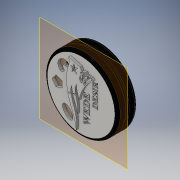
# Autodesk Inventor part: Wheel
Saved by Autodesk Inventor 2016 (Build 200138000, 138)
## iProperties
Created: 2016-10-07
Part Number: Wheel
Material: Generic
Document SubType Name: Modeling
Designer: desirw
Density: 1 g/cm^3
Appearance: Default
Mass: 52.9378 g
Surface Area: 147.304 cm^2
Volume: 52.9378 cm^3
Author: desirw
Autodesk Inventor part; units mm, degrees
ref_plane "YZ Plane" through (0, 0, 0) normal (1, 0, 0) x (0, 1, 0)
ref_plane "XZ Plane" through (0, 0, 0) normal (0, 1, 0) x (-1, 0, 0)
ref_plane "XY Plane" through (0, 0, 0) normal (0, 0, 1) x (1, 0, 0)
sketch "Sketch1" plane through (0, 0, 0) normal (0, 0, 1) x (1, 0, 0)
  circle A0 centre (0, 0) radius 31.75
  dimension "d0" = 63.5
  constraints: 1 centre point, 1 coincident
  measures "d0" diameter of A0
extrude "Extrusion1" add sketch "Sketch1" along normal blind 3.2512
sketch "Sketch2" plane through (0, 0, 3.2512) normal (0, 0, 1) x (1, 0, 0)
  circle A0 centre (0, 0) radius 33.655
  circle A1 centre (0, 0) radius 31.511
  circle A2 centre (0, 0) radius 31.511
  dimension "d3" = 67.31
  dimension "d40" = 2.144
  constraints: 3 centre point, 1 coincident
  measures "d3" diameter of A0
  measures "d40" radial gap between concentric circles of A1 A0
extrude "Extrusion2" add sketch "Sketch2" along normal blind 7.62 contours A0 | A1
sketch "Sketch3" plane through (0, 0, 0) normal (0, 0, -1) x (-1, 0, 0)
  circle A0 centre (0, 0) radius 33.655
  dimension "d6" = 67.31
  constraints: 1 centre point, 1 coincident
  measures "d6" diameter of A0
fillet "Fillet1" radius 2.54 1 edges at (-33.655, 0, 10.8712)
extrude "Extrusion3" add sketch "Sketch3" along normal blind 7.62
fillet "Fillet2" radius 2.54 1 edges at (33.655, 0, -7.62)
sketch "Sketch4" plane through (0, 0, -7.62) normal (0, 0, -1) x (-1, 0, 0)
  arc A0 (1.5256, -7.6067) -> (-1.5256, -7.6067) centre (0, -8.5367) ccw
  line L0 (1.5256, -7.6067) -> (10.0877, -14.0155)
  arc A1 (10.0877, -14.0155) -> (14.0155, -10.0877) centre (11.7691, -11.7691) ccw
  line L1 (14.0155, -10.0877) -> (7.6067, -1.5256)
  arc A2 (7.6067, 1.5256) -> (7.6067, -1.5256) centre (8.5367, 0) ccw
  line L2 (7.6067, 1.5256) -> (14.0155, 10.0877)
  arc A3 (14.0155, 10.0877) -> (10.0877, 14.0155) centre (11.7691, 11.7691) ccw
  line L3 (10.0877, 14.0155) -> (1.5256, 7.6067)
  arc A4 (-1.5256, 7.6067) -> (1.5256, 7.6067) centre (0, 8.5367) ccw
  line L4 (-1.5256, 7.6067) -> (-10.0877, 14.0155)
  arc A5 (-10.0877, 14.0155) -> (-14.0155, 10.0877) centre (-11.7691, 11.7691) ccw
  line L5 (-14.0155, 10.0877) -> (-7.6067, 1.5256)
  arc A6 (-7.6067, -1.5256) -> (-7.6067, 1.5256) centre (-8.5367, 0) ccw
  line L6 (-7.6067, -1.5256) -> (-14.0155, -10.0877)
  arc A7 (-14.0155, -10.0877) -> (-10.0877, -14.0155) centre (-11.7691, -11.7691) ccw
  line L7 (-10.0877, -14.0155) -> (-1.5256, -7.6067)
  circle A8 centre (12.339, -12.339) radius 0.75
  circle A9 centre (9.8641, -9.8641) radius 0.75
  circle A10 centre (7.3893, -7.3893) radius 0.75
  circle A11 centre (4.9144, -4.9144) radius 0.75
  circle A12 centre (12.339, 12.339) radius 0.75
  circle A13 centre (9.8641, 9.8641) radius 0.75
  circle A14 centre (7.3893, 7.3893) radius 0.75
  circle A15 centre (4.9144, 4.9144) radius 0.75
  circle A16 centre (-12.339, 12.339) radius 0.75
  circle A17 centre (-9.8641, 9.8641) radius 0.75
  circle A18 centre (-7.3893, 7.3893) radius 0.75
  circle A19 centre (-4.9144, 4.9144) radius 0.75
  circle A20 centre (-12.339, -12.339) radius 0.75
  circle A21 centre (-9.8641, -9.8641) radius 0.75
  circle A22 centre (-7.3893, -7.3893) radius 0.75
  circle A23 centre (-4.9144, -4.9144) radius 0.75
  circle A24 centre (0, 0) radius 3.6
  constraints: 25 centre point, 16 end point, 16 point on circle
extrude "Extrusion4" cut sketch "Sketch4" against normal blind 2.3622 contours A0 L7 A7 L6 A6 L5 A5 L4 A4 L3 A3 L2 A2 L1 A1 L0 | A8 | A9 | A10 | A11 | A12 | A13 | A14 | A15 | A16 | A17 | A18 | A19 | A20 | A21 | A22 | A23 | A24
sketch "Sketch5" plane through (0, 0, -7.62) normal (0, 0, -1) x (-1, 0, 0)
  circle A0 centre (0, 0) radius 3.6195
  dimension "d15" = 7.239
  constraints: 1 centre point, 1 coincident
  measures "d15" diameter of A0
extrude "Extrusion5" cut sketch "Sketch5" against normal blind 1.1684
sketch "Sketch6" plane through (0, 0, -5.2578) normal (0, 0, -1) x (-1, 0, 0)
  circle A0 centre (0, 0) radius 1.2446
  dimension "d16" = 2.4892
  constraints: 1 centre point, 1 coincident
  measures "d16" diameter of A0
extrude "Extrusion6" cut sketch "Sketch6" against normal blind 7.62
sketch "Sketch7" plane through (0, 0, 10.8712) normal (0, 0, 1) x (1, 0, 0)
  circle A0 centre (0, 0) radius 2.54
  dimension "d19" = 5.08
  constraints: 1 centre point, 1 coincident
  measures "d19" diameter of A0
extrude "Extrusion7" cut sketch "Sketch7" against normal blind 15.24
sketch "Sketch12" plane through (0, 0, -5.2578) normal (0, 0, -1) x (-1, 0, 0)
  circle A0 centre (0, 0) radius 3.5498
  circle A1 centre (0, 0) radius 3.6 projected
  dimension "d41" = 7.2
  constraints: 1 centre point, 1 coincident
  measures "d41" diameter of A1
extrude "Extrusion11" cut sketch "Sketch12" against normal blind 0.508 contours A0
sketch "Sketch13" plane through (0, 0, -7.62) normal (0, 0, -1) x (-1, 0, 0)
  circle A0 centre (-9.8641, -9.8641) radius 1.0795
  circle A1 centre (-9.8641, 9.8641) radius 1.0795
  circle A2 centre (9.8641, 9.8641) radius 1.0795
  circle A3 centre (9.8641, -9.8641) radius 1.0795
  dimension "d46" = 2.159
  dimension "d48" = 2.159
  dimension "d49" = 2.159
  dimension "d50" = 2.159
  constraints: 4 centre point
  measures "d46" diameter of A0
  measures "d48" diameter of A2
  measures "d49" diameter of A3
  measures "d50" diameter of A1
extrude "Extrusion12" cut sketch "Sketch13" against normal blind 50.8
sketch "Sketch16" plane through (0, 0, 10.8712) normal (0, 0, 1) x (1, 0, 0)
  circle A0 centre (0, 0) radius 31.115 projected
  circle A1 centre (0, 0) radius 2.54 projected
  circle A2 centre (0, 0) radius 31.115
  constraints: 1 centre point, 1 coincident, 1 concentric
extrude "Extrusion13" cut sketch "Sketch16" against normal blind 2.54
sketch "Sketch17" plane through (0, 0, 8.3312) normal (0, 0, 1) x (1, 0, 0)
  circle A0 centre (0, 0) radius 1.2446 projected
  circle A1 centre (0, 0) radius 7.62
  circle A2 centre (0, 0) radius 29.21
  dimension "d56" = 15.24
  dimension "d60" = 58.42
  constraints: 2 centre point, 2 coincident
  measures "d56" diameter of A1
  measures "d60" diameter of A2
extrude "Extrusion14" cut sketch "Sketch17" against normal blind 12.7 contours A2
fillet "Fillet3" radius 3.175 2 edges at (-29.21, 0, 8.3312) (-7.62, 0, 8.3312)
sketch "Sketch20" plane through (0, 0, -7.62) normal (0, 0, -1) x (-1, 0, 0)
  circle A0 centre (19.0012, 0) radius 8.4433
  circle A1 centre (0, 0) radius 1.2446 projected
  circle A2 centre (0, 0) radius 2.54 projected
  circle A3 centre (0, -19.0012) radius 8.4433
  circle A4 centre (-19.0012, 0) radius 8.4433
  circle A5 centre (0, 19.0012) radius 8.4433
  arc A6 (15.9108, 14.6269) -> (13.5038, 17.0339) centre (16.1061, 17.2292) ccw construction
  arc A7 (15.8105, 13.2894) -> (12.1662, 16.9336) centre (16.1061, 17.2292) ccw
  arc A8 (16.0112, 15.9644) -> (14.8413, 17.1343) centre (16.1061, 17.2292) ccw
  arc A9 (16.0112, 15.9644) -> (15.8105, 13.2894) centre (15.9108, 14.6269) ccw
  arc A10 (12.1662, 16.9336) -> (14.8413, 17.1343) centre (13.5038, 17.0339) ccw
  arc A11 (14.6269, -15.9108) -> (17.0339, -13.5038) centre (17.2292, -16.1061) ccw construction
  arc A12 (13.2894, -15.8105) -> (16.9336, -12.1662) centre (17.2292, -16.1061) ccw
  arc A13 (15.9644, -16.0112) -> (17.1343, -14.8413) centre (17.2292, -16.1061) ccw
  arc A14 (15.9644, -16.0112) -> (13.2894, -15.8105) centre (14.6269, -15.9108) ccw
  arc A15 (16.9336, -12.1662) -> (17.1343, -14.8413) centre (17.0339, -13.5038) ccw
  arc A16 (-15.9108, -14.6269) -> (-13.5038, -17.0339) centre (-16.1061, -17.2292) ccw construction
  arc A17 (-15.8105, -13.2894) -> (-12.1662, -16.9336) centre (-16.1061, -17.2292) ccw
  arc A18 (-16.0112, -15.9644) -> (-14.8413, -17.1343) centre (-16.1061, -17.2292) ccw
  arc A19 (-16.0112, -15.9644) -> (-15.8105, -13.2894) centre (-15.9108, -14.6269) ccw
  arc A20 (-12.1662, -16.9336) -> (-14.8413, -17.1343) centre (-13.5038, -17.0339) ccw
  arc A21 (-14.6269, 15.9108) -> (-17.0339, 13.5038) centre (-17.2292, 16.1061) ccw construction
  arc A22 (-13.2894, 15.8105) -> (-16.9336, 12.1662) centre (-17.2292, 16.1061) ccw
  arc A23 (-15.9644, 16.0112) -> (-17.1343, 14.8413) centre (-17.2292, 16.1061) ccw
  arc A24 (-15.9644, 16.0112) -> (-13.2894, 15.8105) centre (-14.6269, 15.9108) ccw
  arc A25 (-16.9336, 12.1662) -> (-17.1343, 14.8413) centre (-17.0339, 13.5038) ccw
  dimension "d66" = 360
  dimension "d70" = 360
  constraints: 40 point on circle, 24 centre point, 4 coincident, 4 tangent, 67 other
extrude "Extrusion15" cut sketch "Sketch20" against normal blind 10.16 contours A0 | A3 | A4 | A5 | A9 A8 A10 A7 | A14 A13 A15 A12 | A19 A18 A20 A17 | A24 A23 A25 A22
sketch "Sketch21" plane through (0, 0, -4.3688) normal (0, 0, 1) x (1, 0, 0)
  circle A0 centre (-9.8653, -9.893) radius 2.159
  circle A1 centre (-9.8653, 9.8376) radius 2.159
  circle A2 centre (9.867, -9.893) radius 2.159
  circle A3 centre (9.867, 9.8376) radius 2.159
  point P0 (0, 0)
  dimension "d74" = 4.318
  dimension "d75" = 4.318
  dimension "d76" = 4.318
  dimension "d77" = 4.318
  constraints: 4 centre point
  measures "d74" diameter of A0
  measures "d75" diameter of A1
  measures "d76" diameter of A2
  measures "d77" diameter of A3
extrude "Extrusion16" cut sketch "Sketch21" against normal blind 0.254
sketch "Sketch23" plane through (0, 0, 8.3312) normal (0, 0, 1) x (1, 0, 0)
  circle A0 centre (0, 0) radius 8.0486
  constraints: 1 centre point, 1 coincident
extrude "Extrusion17" cut sketch "Sketch23" against normal blind 12.7
ref_plane "Work Plane2" through (0, 0, 8.3312) normal (0, 0, 1) x (1, 0, 0)
sketch "Sketch24" plane through (0, 0, 8.3312) normal (0, 0, 1) x (1, 0, 0)
  circle A0 centre (0, 0) radius 31.1534
  constraints: 1 centre point, 1 coincident
extrude "Extrusion18" add sketch "Sketch24" along normal blind 2.54
sketch "Sketch25" plane through (0, 0, 10.8712) normal (0, 0, 1) x (1, 0, 0)
  line L0 (-12.7986, -29.9392) -> (-12.7986, 28.2876) construction
  line L1 (-12.7986, 28.2876) -> (14.4515, 28.2876) construction
  line L2 (14.4515, 28.2876) -> (14.4515, -29.9392) construction
  line L3 (14.4515, -29.9392) -> (-12.7986, -29.9392) construction
  arc A0 (-2.4703, -28.2892) -> (-5.6682, -15.7345) centre (-39.8581, -31.1279) ccw
  arc A1 (-10.3026, -1.9948) -> (-5.6682, -15.7345) centre (146.9864, 43.407) ccw
  arc A2 (-2.4703, -28.2892) -> (-2.4703, -18.2629) centre (-33.8456, -23.2761) ccw
  arc A3 (-2.4703, -18.2629) -> (-5.2168, -8.4433) centre (-79.7357, -34.5801) ccw
  arc A4 (-7.0459, -1.252) -> (-5.2168, -8.4433) centre (32.2007, 4.9019) ccw
  line L4 (-10.3026, -1.9948) -> (-7.0459, -1.252)
  arc A5 (-1.4091, -14.8666) -> (-3.8781, -5.8135) centre (-42.9348, -21.3286) ccw
  arc A6 (-5.6682, -0.6984) -> (-3.8781, -5.8135) centre (38.7717, 11.9828) ccw
  arc A7 (-2.9605, 0) -> (-5.6682, -0.6984) centre (0.5008, -19.0171) ccw
  arc A8 (-1.7257, -5.5998) -> (-2.9605, 0) centre (-46.1597, -12.462) ccw
  arc A9 (-1.4091, -14.8666) -> (-1.7257, -5.5998) centre (-31.0492, -11.2405) ccw
  arc A10 (13.0542, 18.6707) -> (0.223, -3.0699) centre (34.2938, -8.5214) ccw
  arc A11 (13.0542, 18.6707) -> (11.4718, 20.2531) centre (10.1474, 17.3464) ccw
  arc A12 (11.4718, 20.2531) -> (9.4266, 20.0581) centre (10.5991, 18.5838) ccw
  arc A13 (9.4266, 20.0581) -> (8.2975, 20.459) centre (7.7468, 17.1172) ccw
  arc A14 (8.2975, 20.459) -> (7.2209, 20.5419) centre (7.4283, 16.2053) ccw
  arc A15 (6.4262, 22.0118) -> (7.2209, 20.5419) centre (11.9084, 24.0263) ccw
  arc A16 (2.6562, 21.2483) -> (6.4262, 22.0118) centre (-20.9306, 147.4079) ccw
  arc A17 (2.6562, 21.2483) -> (1.1935, 24.0263) centre (-252.5291, -111.3406) ccw
  arc A18 (1.1935, 24.0263) -> (-9.4849, 27.0616) centre (-900.7825, -3128.8756) ccw
  arc A19 (-9.1238, 22.0118) -> (-9.4849, 27.0616) centre (-21.4008, 23.6716) ccw
  arc A20 (-10.3026, 17.8312) -> (-9.1238, 22.0118) centre (-36.152, 27.3765) ccw
  arc A21 (-10.3026, 17.8312) -> (-11.3285, 12.6153) centre (170.6673, -20.4736) ccw
  arc A22 (-11.3285, 12.6153) -> (-10.3026, -1.252) centre (38.6762, 9.3432) ccw
  arc A23 (-7.374, -0.5894) -> (-10.3026, -1.252) centre (0.434, -41.9034) ccw
  arc A24 (-6.6405, 5.393) -> (-7.374, -0.5894) centre (2.9307, 1.1832) ccw
  arc A25 (-6.6405, 5.393) -> (-5.8275, -0.1263) centre (42.4689, 9.8072) ccw
  arc A26 (-3.1357, 0.5919) -> (-5.8275, -0.1263) centre (0.6817, -19.118) ccw
  arc A27 (-2.2091, 8.7203) -> (-3.1357, 0.5919) centre (7.8506, 3.4565) ccw
  arc A28 (-2.2091, 8.7203) -> (-1.4091, 2.4558) centre (41.2883, 11.0914) ccw
  arc A29 (0.223, -3.0699) -> (-1.4091, 2.4558) centre (-65.3016, -19.4203) ccw
  arc A30 (6.7707, 15.7398) -> (4.847, 15.3673) centre (16.1173, -37.684) ccw
  arc A31 (4.847, 15.3673) -> (2.5284, 11.9828) centre (51.1574, -18.8455) ccw
  arc A32 (2.0647, 12.0311) -> (2.5284, 11.9828) centre (2.3182, 12.2154) ccw
  arc A33 (0.6817, 14.3084) -> (2.0647, 12.0311) centre (3.8781, 14.6909) ccw
  arc A34 (1.0059, 16.9464) -> (0.6817, 14.3084) centre (8.9448, 14.6319) ccw
  arc A35 (1.507, 17.4809) -> (1.0059, 16.9464) centre (1.5569, 16.9319) ccw
  arc A36 (1.507, 17.4809) -> (1.791, 15.7398) centre (3.5637, 16.9227) ccw
  arc A37 (1.791, 15.7398) -> (2.9878, 14.8708) centre (3.5637, 16.9227) ccw
  line L5 (2.9878, 14.8708) -> (2.9878, 18.3662)
  arc A38 (1.4604, 19.4854) -> (2.9878, 18.3662) centre (3.1078, 20.1318) ccw
  arc A39 (1.3568, 19.6561) -> (1.4604, 19.4854) centre (1.5862, 19.6786) ccw
  arc A40 (1.3568, 20.1992) -> (1.3568, 19.6561) centre (2.2724, 19.9277) ccw
  arc A41 (5.9606, 21.1505) -> (1.3568, 20.1992) centre (8.9783, -5.0691) ccw
  line L6 (5.9606, 21.1505) -> (5.9606, 18.988)
  arc A42 (5.9606, 18.988) -> (6.2957, 18.7748) centre (9.575, 24.2979) ccw
  arc A43 (6.2957, 18.7748) -> (6.9567, 19.9277) centre (-103.158, 82.2966) ccw
  arc A44 (7.5209, 19.9277) -> (6.9567, 19.9277) centre (7.2388, 19.3131) ccw
  line L7 (7.5209, 19.9277) -> (7.5209, 18.6986)
  arc A45 (8.344, 17.7097) -> (7.5209, 18.6986) centre (6.084, 16.6658) ccw
  arc A46 (8.344, 17.7097) -> (8.1842, 18.8788) centre (6.4633, 18.0481) ccw
  line L8 (8.1842, 18.8788) -> (8.1842, 20.0692)
  line L9 (8.1842, 20.0692) -> (8.4773, 20.0692)
  arc A47 (9.1501, 19.6561) -> (8.4773, 20.0692) centre (8.1291, 18.7477) ccw
  line L10 (9.1501, 19.6561) -> (9.1501, 18.878)
  arc A48 (10.3252, 19.7825) -> (9.1501, 18.878) centre (11.157, 17.4862) ccw
  line L11 (10.3252, 19.7825) -> (10.9883, 19.7825)
  arc A49 (12.0805, 18.8788) -> (10.9883, 19.7825) centre (10.1284, 17.6314) ccw
  arc A50 (12.0805, 18.8788) -> (5.0259, 10.9955) centre (36.9587, -10.4824) ccw
  arc A51 (4.3066, 11.9036) -> (5.0259, 10.9955) centre (5.7027, 12.2705) ccw
  arc A52 (4.3066, 12.6373) -> (4.3066, 11.9036) centre (5.7027, 12.2705) ccw
  arc A53 (6.7707, 15.7398) -> (4.3066, 12.6373) centre (9.0478, 11.4015) ccw
  line L12 (-3.2282, 19.8186) -> (-2.0723, 16.5796)
  line L13 (-2.0723, 16.5796) -> (-4.5876, 18.4941)
  line L14 (-4.5876, 18.4941) -> (-6.5126, 16.6185)
  line L15 (-6.5126, 16.6185) -> (-5.8751, 19.474)
  line L16 (-5.8751, 19.474) -> (-7.5613, 20.8788)
  line L17 (-7.5613, 20.8788) -> (-5.366, 21.4271)
  line L18 (-5.366, 21.4271) -> (-4.6252, 24.0672)
  line L19 (-4.6252, 24.0672) -> (-3.8073, 21.7551)
  line L20 (-3.8073, 21.7551) -> (-0.8504, 22.1353)
  line L21 (-0.8504, 22.1353) -> (-3.2282, 19.8186)
  point P0 (0, 0)
  constraints: 110 point on circle, 54 centre point, 36 end point, 5 vertical, 3 concentric, 2 point on line, 1 collinear, 1 horizontal, 1 perpendicular, 2 other
extrude "Extrusion19" add sketch "Sketch25" along normal blind 2.032
sketch "Sketch26" plane through (0, 0, 10.8712) normal (0, 0, 1) x (1, 0, 0)
  line L0 (2.4081, -21.6467) -> (2.4081, -11.4793) construction
  line L1 (2.4081, -11.4793) -> (22.0061, -11.4793) construction
  line L2 (22.0061, -11.4793) -> (22.0061, -21.6467) construction
  line L3 (22.0061, -21.6467) -> (2.4081, -21.6467) construction
  line L4 (10.6883, -4.4342) -> (10.7134, 16.181) construction
  line L5 (10.7134, 16.181) -> (15.654, 16.175) construction
  line L6 (15.654, 16.175) -> (15.6288, -4.4402) construction
  line L7 (15.6288, -4.4402) -> (10.6883, -4.4342) construction
  line L8 (2.4081, -13.0738) -> (2.5626, -13.0738)
  spline S0 degree 2 poles (2.5626, -13.0738) (2.5767, -13.233) (2.7265, -13.453) (2.8857, -13.5373) knots 0 0 0 1 2 2 2
  spline S1 degree 2 poles (2.8857, -13.5373) (2.9372, -13.5607) (3.5412, -13.7995) knots 0 0 0 1 1 1
  line L9 (3.5412, -13.7995) -> (8.2701, -15.5974)
  line L10 (8.2701, -15.5974) -> (8.2701, -15.7613)
  line L11 (8.2701, -15.7613) -> (4.5572, -17.18)
  line L12 (4.5572, -17.18) -> (8.2701, -18.7438)
  line L13 (8.2701, -18.7438) -> (8.2701, -18.8983)
  line L14 (8.2701, -18.8983) -> (3.588, -20.7852)
  spline S2 degree 2 poles (3.588, -20.7852) (2.8857, -21.0708) (2.586, -21.3002) (2.5626, -21.5718) knots 0 0 0 1 2 2 2
  line L15 (2.5626, -21.5718) -> (2.4081, -21.5718)
  line L16 (2.4081, -21.5718) -> (2.4081, -19.0902)
  line L17 (2.4081, -19.0902) -> (2.5626, -19.0902)
  spline S3 degree 2 poles (2.5626, -19.0902) (2.572, -19.3899) (2.7358, -19.5865) (2.8576, -19.5865) knots 0 0 0 1 2 2 2
  spline S4 degree 2 poles (2.8576, -19.5865) (3.0215, -19.5865) (3.5412, -19.3805) knots 0 0 0 1 1 1
  line L18 (3.5412, -19.3805) -> (6.3223, -18.2568)
  line L19 (6.3223, -18.2568) -> (4.1452, -17.3532)
  line L20 (4.1452, -17.3532) -> (3.5412, -17.5873)
  spline S5 degree 2 poles (3.5412, -17.5873) (3.0402, -17.7839) (2.7078, -17.9946) (2.5626, -18.2662) (2.5626, -18.5331) knots 0 0 0 1 2 3 3 3
  line L21 (2.5626, -18.5331) -> (2.4081, -18.5331)
  line L22 (2.4081, -18.5331) -> (2.4081, -15.7613)
  line L23 (2.4081, -15.7613) -> (2.5626, -15.7613)
  spline S6 degree 2 poles (2.5626, -15.7613) (2.5673, -16.0563) (2.6094, -16.1827) knots 0 0 0 1 1 1
  spline S7 degree 2 poles (2.6094, -16.1827) (2.6375, -16.2716) (2.778, -16.37) (2.8669, -16.37) knots 0 0 0 1 2 2 2
  spline S8 degree 2 poles (2.8669, -16.37) (2.9653, -16.37) (3.4663, -16.1827) knots 0 0 0 1 1 1
  line L24 (3.4663, -16.1827) -> (6.1772, -15.1386)
  line L25 (6.1772, -15.1386) -> (3.7238, -14.2021)
  spline S9 degree 2 poles (3.7238, -14.2021) (3.3398, -14.057) (3.0636, -13.9868) (2.9419, -13.9868) knots 0 0 0 1 2 2 2
  spline S10 degree 2 poles (2.9419, -13.9868) (2.7686, -13.9868) (2.572, -14.2256) (2.5626, -14.558) knots 0 0 0 1 2 2 2
  line L26 (2.5626, -14.558) -> (2.4081, -14.558)
  line L27 (2.4081, -14.558) -> (2.4081, -13.0738)
  line L28 (2.7358, -10.6344) -> (5.0675, -10.6344)
  line L29 (5.0675, -10.6344) -> (5.0675, -10.5173)
  spline S11 degree 2 poles (5.0675, -10.5173) (5.0675, -9.9695) (4.3839, -9.4779) (3.7144, -9.4077) knots 0 0 0 1 2 2 2
  line L30 (3.7144, -9.4077) -> (3.7144, -9.2532)
  line L31 (3.7144, -9.2532) -> (6.7156, -9.2532)
  line L32 (6.7156, -9.2532) -> (6.7156, -9.4077)
  spline S12 degree 2 poles (6.7156, -9.4077) (6.224, -9.4592) (5.6013, -9.7869) (5.3859, -10.2224) (5.3859, -10.6344) knots 0 0 0 1 2 3 3 3
  line L33 (5.3859, -10.6344) -> (7.0012, -10.6344)
  spline S13 degree 2 poles (7.0012, -10.6344) (7.4741, -10.6344) (7.6848, -10.5548) (7.8206, -10.3347) (7.8206, -10.0866) knots 0 0 0 1 2 3 3 3
  line L34 (7.8206, -10.0866) -> (7.8206, -9.7448)
  spline S14 degree 2 poles (7.8206, -9.7448) (7.8206, -8.9395) (7.0761, -7.9703) (6.3176, -7.7596) knots 0 0 0 1 2 2 2
  line L35 (6.3176, -7.7596) -> (6.3176, -7.6051)
  line L36 (6.3176, -7.6051) -> (8.139, -7.8626)
  line L37 (8.139, -7.8626) -> (8.139, -12.8162)
  line L38 (8.139, -12.8162) -> (7.9845, -12.8162)
  line L39 (7.9845, -12.8162) -> (7.9845, -12.6243)
  spline S15 degree 2 poles (7.9845, -12.6243) (7.9845, -12.3761) (7.8955, -12.2263) knots 0 0 0 1 1 1
  spline S16 degree 2 poles (7.8955, -12.2263) (7.8346, -12.1186) (7.6942, -12.0578) knots 0 0 0 1 1 1
  spline S17 degree 2 poles (7.6942, -12.0578) (7.5912, -12.0109) (7.1604, -12.0109) knots 0 0 0 1 1 1
  line L40 (7.1604, -12.0109) -> (3.3867, -12.0109)
  spline S18 degree 2 poles (3.3867, -12.0109) (2.998, -12.0109) (2.9091, -12.0297) knots 0 0 0 1 1 1
  spline S19 degree 2 poles (2.9091, -12.0297) (2.7593, -12.0765) (2.6797, -12.1888) knots 0 0 0 1 1 1
  spline S20 degree 2 poles (2.6797, -12.1888) (2.5626, -12.348) (2.5626, -12.6243) knots 0 0 0 1 1 1
  line L41 (2.5626, -12.6243) -> (2.5626, -12.8162)
  line L42 (2.5626, -12.8162) -> (2.4081, -12.8162)
  line L43 (2.4081, -12.8162) -> (2.4081, -8.0171)
  line L44 (2.4081, -8.0171) -> (4.103, -8.0171)
  line L45 (4.103, -8.0171) -> (4.103, -8.1716)
  spline S21 degree 2 poles (4.103, -8.1716) (3.4803, -8.2934) (2.9372, -8.7428) (2.8108, -9.1502) knots 0 0 0 1 2 2 2
  spline S22 degree 2 poles (2.8108, -9.1502) (2.7358, -9.3843) (2.7358, -10.0398) knots 0 0 0 1 1 1
  line L46 (2.7358, -10.0398) -> (2.7358, -10.6344)
  line L47 (8.139, -7.0994) -> (7.9845, -7.0994)
  line L48 (7.9845, -7.0994) -> (7.9845, -6.9075)
  spline S23 degree 2 poles (7.9845, -6.9075) (7.9845, -6.6593) (7.83, -6.3971) (7.6942, -6.3316) knots 0 0 0 1 2 2 2
  spline S24 degree 2 poles (7.6942, -6.3316) (7.6052, -6.2941) (7.1604, -6.2941) knots 0 0 0 1 1 1
  line L49 (7.1604, -6.2941) -> (3.3867, -6.2941)
  spline S25 degree 2 poles (3.3867, -6.2941) (2.9465, -6.2941) (2.7265, -6.3877) (2.5626, -6.6687) (2.5626, -6.9075) knots 0 0 0 1 2 3 3 3
  line L50 (2.5626, -6.9075) -> (2.5626, -7.0994)
  line L51 (2.5626, -7.0994) -> (2.4081, -7.0994)
  line L52 (2.4081, -7.0994) -> (2.4081, -4.5383)
  spline S26 degree 2 poles (2.4081, -4.5383) (2.4081, -3.5083) (2.689, -2.8855) knots 0 0 0 1 1 1
  spline S27 degree 2 poles (2.689, -2.8855) (3.0308, -2.1224) (4.4167, -1.3311) (5.2923, -1.3311) knots 0 0 0 1 2 2 2
  spline S28 degree 2 poles (5.2923, -1.3311) (5.8963, -1.3311) (6.9123, -1.7197) (7.5771, -2.3377) (7.9798, -3.1431) (8.0875, -3.7236) knots 0 0 0 1 2 3 4 4 4
  spline S29 degree 2 poles (8.0875, -3.7236) (8.139, -3.9812) (8.139, -4.5383) knots 0 0 0 1 1 1
  line L53 (8.139, -4.5383) -> (8.139, -7.0994)
  line L54 (2.7358, -4.9176) -> (7.2026, -4.9176)
  spline S30 degree 2 poles (7.2026, -4.9176) (7.5537, -4.9176) (7.7129, -4.852) (7.755, -4.7677) knots 0 0 0 1 2 2 2
  spline S31 degree 2 poles (7.755, -4.7677) (7.8206, -4.6554) (7.8206, -4.44) knots 0 0 0 1 1 1
  spline S32 degree 2 poles (7.8206, -4.44) (7.8206, -3.7377) (7.3383, -3.3631) knots 0 0 0 1 1 1
  spline S33 degree 2 poles (7.3383, -3.3631) (6.6875, -2.8575) (5.3204, -2.8575) knots 0 0 0 1 1 1
  spline S34 degree 2 poles (5.3204, -2.8575) (4.2201, -2.8575) (3.5646, -3.2039) knots 0 0 0 1 1 1
  spline S35 degree 2 poles (3.5646, -3.2039) (3.0495, -3.4802) (2.8623, -3.9109) knots 0 0 0 1 1 1
  spline S36 degree 2 poles (2.8623, -3.9109) (2.7312, -4.2106) (2.7358, -4.9176) knots 0 0 0 1 1 1
  line L55 (2.7358, 1.3892) -> (5.0675, 1.3892)
  line L56 (5.0675, 1.3892) -> (5.0675, 1.5063)
  spline S37 degree 2 poles (5.0675, 1.5063) (5.0675, 2.0541) (4.3839, 2.5457) (3.7144, 2.6159) knots 0 0 0 1 2 2 2
  line L57 (3.7144, 2.6159) -> (3.7144, 2.7704)
  line L58 (3.7144, 2.7704) -> (6.7156, 2.7704)
  line L59 (6.7156, 2.7704) -> (6.7156, 2.6159)
  spline S38 degree 2 poles (6.7156, 2.6159) (6.224, 2.5644) (5.6013, 2.2367) (5.3859, 1.8012) (5.3859, 1.3892) knots 0 0 0 1 2 3 3 3
  line L60 (5.3859, 1.3892) -> (7.0012, 1.3892)
  spline S39 degree 2 poles (7.0012, 1.3892) (7.4741, 1.3892) (7.6848, 1.4688) (7.8206, 1.6889) (7.8206, 1.937) knots 0 0 0 1 2 3 3 3
  line L61 (7.8206, 1.937) -> (7.8206, 2.2788)
  spline S40 degree 2 poles (7.8206, 2.2788) (7.8206, 3.0841) (7.0761, 4.0533) (6.3176, 4.264) knots 0 0 0 1 2 2 2
  line L62 (6.3176, 4.264) -> (6.3176, 4.4185)
  line L63 (6.3176, 4.4185) -> (8.139, 4.161)
  line L64 (8.139, 4.161) -> (8.139, -0.7926)
  line L65 (8.139, -0.7926) -> (7.9845, -0.7926)
  line L66 (7.9845, -0.7926) -> (7.9845, -0.6007)
  spline S41 degree 2 poles (7.9845, -0.6007) (7.9845, -0.3525) (7.8955, -0.2027) knots 0 0 0 1 1 1
  spline S42 degree 2 poles (7.8955, -0.2027) (7.8346, -0.095) (7.6942, -0.0342) knots 0 0 0 1 1 1
  spline S43 degree 2 poles (7.6942, -0.0342) (7.5912, 0.0127) (7.1604, 0.0127) knots 0 0 0 1 1 1
  line L67 (7.1604, 0.0127) -> (3.3867, 0.0127)
  spline S44 degree 2 poles (3.3867, 0.0127) (2.998, 0.0127) (2.9091, -0.0061) knots 0 0 0 1 1 1
  spline S45 degree 2 poles (2.9091, -0.0061) (2.7593, -0.0529) (2.6797, -0.1653) knots 0 0 0 1 1 1
  spline S46 degree 2 poles (2.6797, -0.1653) (2.5626, -0.3244) (2.5626, -0.6007) knots 0 0 0 1 1 1
  line L68 (2.5626, -0.6007) -> (2.5626, -0.7926)
  line L69 (2.5626, -0.7926) -> (2.4081, -0.7926)
  line L70 (2.4081, -0.7926) -> (2.4081, 4.0065)
  line L71 (2.4081, 4.0065) -> (4.103, 4.0065)
  line L72 (4.103, 4.0065) -> (4.103, 3.852)
  spline S47 degree 2 poles (4.103, 3.852) (3.4803, 3.7302) (2.9372, 3.2808) (2.8108, 2.8734) knots 0 0 0 1 2 2 2
  spline S48 degree 2 poles (2.8108, 2.8734) (2.7358, 2.6393) (2.7358, 1.9838) knots 0 0 0 1 1 1
  line L73 (2.7358, 1.9838) -> (2.7358, 1.3892)
  line L74 (15.5208, -4.3436) -> (15.3935, -4.3435)
  line L75 (15.3935, -4.3435) -> (15.3937, -4.1852)
  spline S49 degree 2 poles (15.3937, -4.1852) (15.3939, -3.9806) (15.2668, -3.7643) (15.1549, -3.7102) knots 0 0 0 1 2 2 2
  spline S50 degree 2 poles (15.1549, -3.7102) (15.0816, -3.6792) (14.715, -3.6787) knots 0 0 0 1 1 1
  line L76 (14.715, -3.6787) -> (11.604, -3.6749)
  spline S51 degree 2 poles (11.604, -3.6749) (11.2411, -3.6745) (11.0596, -3.7515) (10.9243, -3.9829) (10.924, -4.1797) knots 0 0 0 1 2 3 3 3
  line L77 (10.924, -4.1797) -> (10.9238, -4.338)
  line L78 (10.9238, -4.338) -> (10.7964, -4.3378)
  line L79 (10.7964, -4.3378) -> (10.799, -2.2265)
  spline S52 degree 2 poles (10.799, -2.2265) (10.8001, -1.3774) (11.0323, -0.8643) knots 0 0 0 1 1 1
  spline S53 degree 2 poles (11.0323, -0.8643) (11.3148, -0.2355) (12.4581, 0.4154) (13.1799, 0.4145) knots 0 0 0 1 2 2 2
  spline S54 degree 2 poles (13.1799, 0.4145) (13.6778, 0.4139) (14.515, 0.0925) (15.0625, -0.4176) (15.3936, -1.0819) (15.4818, -1.5606) knots 0 0 0 1 2 3 4 4 4
  spline S55 degree 2 poles (15.4818, -1.5606) (15.524, -1.773) (15.5234, -2.2323) knots 0 0 0 1 1 1
  line L80 (15.5234, -2.2323) -> (15.5208, -4.3436)
  line L81 (11.0688, -2.5395) -> (14.7511, -2.544)
  spline S56 degree 2 poles (14.7511, -2.544) (15.0406, -2.5444) (15.1719, -2.4905) (15.2067, -2.421) knots 0 0 0 1 2 2 2
  spline S57 degree 2 poles (15.2067, -2.421) (15.2608, -2.3285) (15.2611, -2.1509) knots 0 0 0 1 1 1
  spline S58 degree 2 poles (15.2611, -2.1509) (15.2618, -1.572) (14.8646, -1.2627) knots 0 0 0 1 1 1
  spline S59 degree 2 poles (14.8646, -1.2627) (14.3286, -0.8452) (13.2015, -0.8438) knots 0 0 0 1 1 1
  spline S60 degree 2 poles (13.2015, -0.8438) (12.2945, -0.8427) (11.7537, -1.1276) knots 0 0 0 1 1 1
  spline S61 degree 2 poles (11.7537, -1.1276) (11.3289, -1.3549) (11.1741, -1.7098) knots 0 0 0 1 1 1
  spline S62 degree 2 poles (11.1741, -1.7098) (11.0657, -1.9567) (11.0688, -2.5395) knots 0 0 0 1 1 1
  line L82 (11.0752, 2.6597) -> (12.9974, 2.6573)
  line L83 (12.9974, 2.6573) -> (12.9975, 2.7538)
  spline S63 degree 2 poles (12.9975, 2.7538) (12.998, 3.2054) (12.435, 3.6114) (11.8831, 3.6699) knots 0 0 0 1 2 2 2
  line L84 (11.8831, 3.6699) -> (11.8833, 3.7973)
  line L85 (11.8833, 3.7973) -> (14.3574, 3.7943)
  line L86 (14.3574, 3.7943) -> (14.3573, 3.6669)
  spline S64 degree 2 poles (14.3573, 3.6669) (13.9519, 3.6249) (13.4382, 3.3554) (13.2602, 2.9966) (13.2598, 2.657) knots 0 0 0 1 2 3 3 3
  line L87 (13.2598, 2.657) -> (14.5915, 2.6554)
  spline S65 degree 2 poles (14.5915, 2.6554) (14.9813, 2.6549) (15.1551, 2.7203) (15.2672, 2.9016) (15.2675, 3.1061) knots 0 0 0 1 2 3 3 3
  line L88 (15.2675, 3.1061) -> (15.2678, 3.3879)
  spline S66 degree 2 poles (15.2678, 3.3879) (15.2686, 4.0518) (14.6559, 4.8515) (14.0308, 5.026) knots 0 0 0 1 2 2 2
  line L89 (14.0308, 5.026) -> (14.031, 5.1533)
  line L90 (14.031, 5.1533) -> (15.5322, 4.9392)
  line L91 (15.5322, 4.9392) -> (15.5272, 0.8555)
  line L92 (15.5272, 0.8555) -> (15.3998, 0.8557)
  line L93 (15.3998, 0.8557) -> (15.4, 1.0139)
  spline S67 degree 2 poles (15.4, 1.0139) (15.4003, 1.2185) (15.3271, 1.3421) knots 0 0 0 1 1 1
  spline S68 degree 2 poles (15.3271, 1.3421) (15.277, 1.431) (15.1613, 1.4813) knots 0 0 0 1 1 1
  spline S69 degree 2 poles (15.1613, 1.4813) (15.0764, 1.52) (14.7213, 1.5204) knots 0 0 0 1 1 1
  line L94 (14.7213, 1.5204) -> (11.6103, 1.5242)
  spline S70 degree 2 poles (11.6103, 1.5242) (11.2899, 1.5246) (11.2166, 1.5093) knots 0 0 0 1 1 1
  spline S71 degree 2 poles (11.2166, 1.5093) (11.093, 1.4708) (11.0273, 1.3783) knots 0 0 0 1 1 1
  spline S72 degree 2 poles (11.0273, 1.3783) (10.9306, 1.2471) (10.9304, 1.0194) knots 0 0 0 1 1 1
  line L95 (10.9304, 1.0194) -> (10.9302, 0.8612)
  line L96 (10.9302, 0.8612) -> (10.8028, 0.8613)
  line L97 (10.8028, 0.8613) -> (10.8076, 4.8176)
  line L98 (10.8076, 4.8176) -> (12.2049, 4.8159)
  line L99 (12.2049, 4.8159) -> (12.2047, 4.6885)
  spline S73 degree 2 poles (12.2047, 4.6885) (11.6913, 4.5888) (11.2431, 4.2188) (11.1384, 3.8831) knots 0 0 0 1 2 2 2
  spline S74 degree 2 poles (11.1384, 3.8831) (11.0764, 3.6902) (11.0758, 3.1498) knots 0 0 0 1 1 1
  line L100 (11.0758, 3.1498) -> (11.0752, 2.6597)
  line L101 (10.7045, 8.8281) -> (12.2793, 8.8647)
  line L102 (12.2793, 8.8647) -> (12.2791, 8.7219)
  spline S75 degree 2 poles (12.2791, 8.7219) (11.6885, 8.6223) (10.9657, 7.8281) (10.9651, 7.3687) knots 0 0 0 1 2 2 2
  spline S76 degree 2 poles (10.9651, 7.3687) (10.9647, 7.0136) (11.3425, 6.5963) (11.5895, 6.596) knots 0 0 0 1 2 2 2
  spline S77 degree 2 poles (11.5895, 6.596) (11.7477, 6.5958) (11.8675, 6.669) knots 0 0 0 1 1 1
  spline S78 degree 2 poles (11.8675, 6.669) (12.0336, 6.7692) (12.1921, 6.9928) knots 0 0 0 1 1 1
  spline S79 degree 2 poles (12.1921, 6.9928) (12.3081, 7.1587) (12.6022, 7.7527) knots 0 0 0 1 1 1
  spline S80 degree 2 poles (12.6022, 7.7527) (13.0085, 8.5821) (13.3716, 8.8711) knots 0 0 0 1 1 1
  spline S81 degree 2 poles (13.3716, 8.8711) (13.7348, 9.1563) (14.2018, 9.1557) knots 0 0 0 1 1 1
  spline S82 degree 2 poles (14.2018, 9.1557) (14.7924, 9.155) (15.6443, 8.2315) (15.6434, 7.5174) knots 0 0 0 1 2 2 2
  spline S83 degree 2 poles (15.6434, 7.5174) (15.6431, 7.2936) (15.5539, 6.8961) (15.4261, 6.5991) knots 0 0 0 1 2 2 2
  spline S84 degree 2 poles (15.4261, 6.5991) (15.3565, 6.4293) (15.3563, 6.3212) knots 0 0 0 1 1 1
  spline S85 degree 2 poles (15.3563, 6.3212) (15.3562, 6.2325) (15.4988, 6.0277) (15.6415, 5.9658) knots 0 0 0 1 2 2 2
  line L103 (15.6415, 5.9658) -> (15.6414, 5.8384)
  line L104 (15.6414, 5.8384) -> (13.8581, 5.8406)
  line L105 (13.8581, 5.8406) -> (13.8583, 5.968)
  spline S86 degree 2 poles (13.8583, 5.968) (14.6111, 6.1214) (15.3996, 6.9966) (15.4002, 7.5023) knots 0 0 0 1 2 2 2
  spline S87 degree 2 poles (15.4002, 7.5023) (15.4007, 7.8921) (14.9767, 8.3558) (14.6949, 8.3562) knots 0 0 0 1 2 2 2
  spline S88 degree 2 poles (14.6949, 8.3562) (14.529, 8.3564) (14.2122, 8.1792) (13.93, 7.8167) (13.7056, 7.3538) knots 0 0 0 1 2 3 3 3
  spline S89 degree 2 poles (13.7056, 7.3538) (13.3883, 6.7096) (12.9399, 6.1466) (12.3914, 5.8462) (12.0595, 5.8466) knots 0 0 0 1 2 3 3 3
  spline S90 degree 2 poles (12.0595, 5.8466) (11.4959, 5.8473) (10.7018, 6.6782) (10.7026, 7.3073) knots 0 0 0 1 2 2 2
  spline S91 degree 2 poles (10.7026, 7.3073) (10.7029, 7.5389) (10.7572, 7.755) knots 0 0 0 1 1 1
  spline S92 degree 2 poles (10.7572, 7.755) (10.7998, 7.917) (11.0281, 8.3877) (11.0283, 8.4842) knots 0 0 0 1 2 2 2
  spline S93 degree 2 poles (11.0283, 8.4842) (11.0284, 8.5729) (10.9166, 8.6773) (10.7043, 8.7239) knots 0 0 0 1 2 2 2
  line L106 (10.7043, 8.7239) -> (10.7045, 8.8281)
  line L107 (15.4135, 12.0453) -> (15.5409, 12.0451)
  line L108 (15.5409, 12.0451) -> (15.5379, 9.5826)
  line L109 (15.5379, 9.5826) -> (15.4105, 9.5827)
  line L110 (15.4105, 9.5827) -> (15.4107, 9.741)
  spline S94 degree 2 poles (15.4107, 9.741) (15.4109, 9.9455) (15.3377, 10.0691) knots 0 0 0 1 1 1
  spline S95 degree 2 poles (15.3377, 10.0691) (15.2877, 10.158) (15.1719, 10.2083) knots 0 0 0 1 1 1
  spline S96 degree 2 poles (15.1719, 10.2083) (15.0871, 10.247) (14.732, 10.2474) knots 0 0 0 1 1 1
  line L111 (14.732, 10.2474) -> (11.621, 10.2512)
  spline S97 degree 2 poles (11.621, 10.2512) (11.2582, 10.2517) (11.0766, 10.1747) (10.9413, 9.9433) (10.941, 9.7464) knots 0 0 0 1 2 3 3 3
  line L112 (10.941, 9.7464) -> (10.9408, 9.5882)
  line L113 (10.9408, 9.5882) -> (10.8135, 9.5883)
  line L114 (10.8135, 9.5883) -> (10.8165, 12.0509)
  line L115 (10.8165, 12.0509) -> (10.9438, 12.0507)
  line L116 (10.9438, 12.0507) -> (10.9437, 11.8963)
  spline S98 degree 2 poles (10.9437, 11.8963) (10.9434, 11.6918) (11.0166, 11.5682) knots 0 0 0 1 1 1
  spline S99 degree 2 poles (11.0166, 11.5682) (11.0667, 11.4755) (11.1824, 11.4251) knots 0 0 0 1 1 1
  spline S100 degree 2 poles (11.1824, 11.4251) (11.2673, 11.3864) (11.6224, 11.386) knots 0 0 0 1 1 1
  line L117 (11.6224, 11.386) -> (14.7334, 11.3822)
  spline S101 degree 2 poles (14.7334, 11.3822) (15.0962, 11.3818) (15.2777, 11.4626) (15.4131, 11.694) (15.4133, 11.8909) knots 0 0 0 1 2 3 3 3
  line L118 (15.4133, 11.8909) -> (15.4135, 12.0453)
  line L119 (13.3896, 14.1166) -> (14.7135, 14.115)
  spline S102 degree 2 poles (14.7135, 14.115) (15.0995, 14.1145) (15.2965, 14.2069) (15.4164, 14.4461) (15.4168, 14.7703) knots 0 0 0 1 2 3 3 3
  line L120 (15.4168, 14.7703) -> (15.5442, 14.7701)
  line L121 (15.5442, 14.7701) -> (15.5412, 12.35)
  line L122 (15.5412, 12.35) -> (15.4139, 12.3502)
  spline S103 degree 2 poles (15.4139, 12.3502) (15.4143, 12.6783) (15.291, 12.9139) (15.0982, 13.0067) (14.7122, 13.0072) knots 0 0 0 1 2 3 3 3
  line L123 (14.7122, 13.0072) -> (11.6475, 13.011)
  spline S104 degree 2 poles (11.6475, 13.011) (11.2615, 13.0114) (11.0646, 12.919) (10.9446, 12.6799) (10.9442, 12.3556) knots 0 0 0 1 2 3 3 3
  line L124 (10.9442, 12.3556) -> (10.8168, 12.3558)
  line L125 (10.8168, 12.3558) -> (10.8195, 14.552)
  spline S105 degree 2 poles (10.8195, 14.552) (10.8206, 15.4089) (11.057, 16.2037) (11.6945, 16.7047) (12.1229, 16.7042) knots 0 0 0 1 2 3 3 3
  spline S106 degree 2 poles (12.1229, 16.7042) (12.6478, 16.7036) (12.987, 16.3249) knots 0 0 0 1 1 1
  spline S107 degree 2 poles (12.987, 16.3249) (13.2029, 16.0853) (13.3104, 15.6529) knots 0 0 0 1 1 1
  line L126 (13.3104, 15.6529) -> (14.9137, 16.7857)
  spline S108 degree 2 poles (14.9137, 16.7857) (15.2266, 17.0092) (15.3, 17.1056) knots 0 0 0 1 1 1
  spline S109 degree 2 poles (15.3, 17.1056) (15.4083, 17.2483) (15.4201, 17.4374) knots 0 0 0 1 1 1
  line L127 (15.4201, 17.4374) -> (15.5475, 17.4372)
  line L128 (15.5475, 17.4372) -> (15.5456, 15.9474)
  line L129 (15.5456, 15.9474) -> (13.39, 14.4254)
  line L130 (13.39, 14.4254) -> (13.3896, 14.1166)
  line L131 (11.0737, 14.1194) -> (13.1426, 14.1169)
  line L132 (13.1426, 14.1169) -> (13.1428, 14.3137)
  spline S110 degree 2 poles (13.1428, 14.3137) (13.1434, 14.8001) (12.9665, 15.2828) (12.5036, 15.5574) (12.1292, 15.5578) knots 0 0 0 1 2 3 3 3
  spline S111 degree 2 poles (12.1292, 15.5578) (11.5927, 15.5585) (11.0749, 15.0535) (11.0742, 14.4938) knots 0 0 0 1 2 2 2
  line L133 (11.0742, 14.4938) -> (11.0737, 14.1194)
  point P0 (0, 0)
  constraints: 4 other
extrude "Extrusion20" cut sketch "Sketch26" against normal blind 7.62
sketch "Sketch28" plane through (0, 0, 10.8712) normal (0, 0, 1) x (1, 0, 0)
  line L0 (-26.6898, -0.1008) -> (-23.2204, 4.6745)
  line L1 (-23.2204, 4.6745) -> (-17.6067, 2.8505)
  line L2 (-17.6067, 2.8505) -> (-17.6067, -3.052)
  line L3 (-17.6067, -3.052) -> (-23.2204, -4.876)
  line L4 (-23.2204, -4.876) -> (-26.6898, -0.1008)
  ellipse E0 centre (-12.3416, -19.2562) end of major axis (-16.3268, -14.3642) minor radius 3.5928
  arc A0 (-13.856, 18.5476) -> (-17.8411, 12.1419) centre (-15.3453, 15.0316) ccw construction
  arc A1 (-12.9756, 20.626) -> (-19.3165, 10.4336) centre (-15.3453, 15.0316) ccw
  arc A2 (-14.7364, 16.4691) -> (-16.3657, 13.8501) centre (-15.3453, 15.0316) ccw
  arc A3 (-14.7364, 16.4691) -> (-12.9756, 20.626) centre (-13.856, 18.5476) ccw
  arc A4 (-19.3165, 10.4336) -> (-16.3657, 13.8501) centre (-17.8411, 12.1419) ccw
  point P0 (-21.6688, -0.1008)
  constraints: 10 end point, 10 point on circle, 5 centre point, 4 tangent, 1 vertical, 13 other
extrude "Extrusion21" cut sketch "Sketch28" against normal blind 7.62
body "Solid1"
